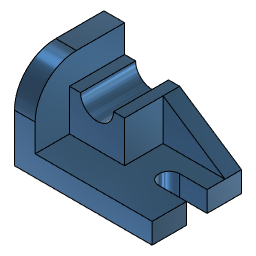
Exercise-6 v1 (Autodesk Fusion 360 design; units mm, degrees)
Autodesk Fusion 360 part; units mm, degrees
sketch "Sketch1" plane through (0, 0, 0) normal (0, 0, 1) x (1, 0, 0)
  line L0 (0, 0) -> (100, 0)
  line L1 (100, 0) -> (100, 65)
  line L2 (100, 65) -> (0, 65)
  line L3 (0, 65) -> (0, 0)
  dimension "d1" = 100
  dimension "d2" = 65
  constraint horizontal L0
  constraint vertical L1
  constraint horizontal L2
  constraint vertical L3
  constraint coincident L0.start L3.end
  measures "d1" distance of L0.start L0.end
  measures "d2" distance of L0.start L2.end
extrude "Extrude1" add sketch "Sketch1" along normal blind 15
sketch "Sketch2" plane through (0, 0, 15) normal (0, 0, 1) x (-1, 0, 0)
  line L0 (0, -65) -> (0, 0)
  line L1 (0, 0) -> (-100, 0)
  line L2 (-100, 0) -> (-100, -65)
  line L3 (-100, -65) -> (0, -65)
  line L4 (0, -65) -> (-15, -65)
  line L5 (-15, -65) -> (-15, 0)
  line L6 (-15, 0) -> (0, 0)
  line L7 (0, 0) -> (0, -65)
  line L8 (-15, -65) -> (-55, -65)
  line L9 (-55, -65) -> (-55, -25)
  line L10 (-55, -25) -> (-15, -25)
  line L11 (-15, -25) -> (-15, -65)
  line L12 (-55, -65) -> (-100, -65)
  line L13 (-100, -65) -> (-100, -53)
  line L14 (-100, -53) -> (-55, -53)
  line L15 (-55, -53) -> (-55, -65)
  line L16 (-80, -40) -> (-100, -40)
  line L17 (-100, -40) -> (-100, -25)
  line L18 (-100, -25) -> (-80, -25)
  arc A0 (-80, -40) -> (-80.003, -25) centre (-80, -32.5) ccw
  dimension "d5" = 15
  dimension "d6" = 65
  dimension "d7" = 40
  dimension "d8" = 40
  dimension "d9" = 45
  dimension "d10" = 12
  dimension "d11" = 15
  dimension "d12" = 20
  dimension "d13" = 20
  dimension "d14" = 15
  constraint horizontal L4
  constraint vertical L5
  constraint horizontal L6
  constraint vertical L7
  constraint coincident L0.start L3.end
  constraint horizontal L8
  constraint vertical L9
  constraint horizontal L10
  constraint vertical L11
  constraint horizontal L12
  constraint vertical L13
  constraint horizontal L14
  constraint vertical L15
  constraint horizontal L16
  constraint vertical L17
  constraint horizontal L18
  constraint coincident L18 A0.end
  measures "d5" distance of L0.start L4.end
  measures "d6" distance of L0.start L0.end
  measures "d7" distance of L4.end L8.end
  measures "d8" distance of L4.end L10.end
  measures "d9" distance of L8.end L2.end
  measures "d10" distance of L8.end L14.end
  measures "d11" diameter of A0
  measures "d12" distance of L2 A0.centre
  measures "d13" distance of L16.start L16.end
  measures "d14" distance of L16.start L18.end
extrude "Extrude2" add sketch "Sketch2" along normal blind 50 contours L0 L1 L3 L4 L5 L6 L7 L11
extrude "Extrude3" add sketch "Sketch2" along normal blind 30 contours L3 L5 L8 L9 L10 L11 L15 | L2 L3 L9 L12 L13 L14 L15
extrude "Extrude4" cut sketch "Sketch2" against normal blind 30 contours L2 L16 L17 L18 A0
sketch "Sketch3" plane through (0, 53, 0) normal (0, -1, 0) x (1, 0, 0)
  line L0 (55, 15) -> (100, 15)
  line L1 (100, 15) -> (100, 45)
  line L2 (100, 45) -> (55, 45)
  line L3 (55, 45) -> (55, 15)
  line L4 (55, 45) -> (100, 15)
  line L5 (100, 45) -> (55, 45)
  line L6 (100, 45) -> (100, 15)
  constraint coincident L2.end L3.start
  constraint coincident L0.end L1.start
  constraint coincident L1.end L2.start
fillet "Fillet1" radius 30 1 edges at (7.5, 0, 65)
sketch "Sketch5" plane through (0, 25, 0) normal (0, -1, 0) x (1, 0, 0)
  line L0 (15, 15) -> (55, 15)
  line L1 (55, 15) -> (55, 45)
  line L2 (55, 45) -> (15, 45)
  line L3 (15, 45) -> (15, 15)
  line L4 (15, 45) -> (23, 45)
  line L5 (55, 45) -> (47, 45)
  line L6 (23, 45) -> (35, 45)
  circle A0 centre (35, 45) radius 12
  dimension "d25" = 8
  dimension "d26" = 8
  dimension "d27" = 12
  dimension "d28" = 24
  constraint coincident L2.end L3.start
  constraint perpendicular L3 L4
  constraint coincident L1.end L2.start
  constraint perpendicular L1 L5
  constraint parallel L2 L6
  constraint coincident L6.end A0.centre
  measures "d25" distance of L2.end L4.end
  measures "d26" distance of L1.end L5.end
  measures "d27" distance of L4.end L6.end
  measures "d28" diameter of A0
chamfer "Chamfer1" distance 45 distance2 30 1 edges at (100, 59, 45) measured on face at (28.3333, 47.6667, 45)
sketch "Sketch6" plane through (0, 0, 45) normal (0, 0, 1) x (-1, 0, 0)
  line L0 (-55, -53) -> (-55, -65)
  line L1 (-55, -65) -> (-15, -65)
  line L2 (-15, -65) -> (-15, -25)
  line L3 (-15, -25) -> (-55, -25)
  line L4 (-55, -25) -> (-55, -53)
  line L5 (-35, -65) -> (-47, -65)
  line L6 (-47, -65) -> (-47, -25)
  line L7 (-47, -25) -> (-35, -25)
  line L8 (-35, -25) -> (-35, -65)
  dimension "d33" = 12
  dimension "d34" = 40
  constraint horizontal L5
  constraint vertical L6
  constraint horizontal L7
  constraint vertical L8
  constraint midpoint L1 L5.start
  measures "d33" distance of L5.start L5.end
  measures "d34" distance of L5.start L7.end
revolve "Revolve1" cut sketch "Sketch6" angle 360 about axis through (35, 25, 45) along (0, 1, 0) contours L1 L3 L5 L6 L7 L8
